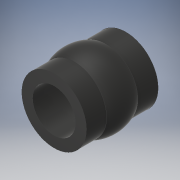
# Autodesk Inventor part: タミヤダンパー部品8.1
Saved by Autodesk Inventor 2020.1 (Build 241239000, 239)
## iProperties
Created: 2018-09-17
Part Number: タミヤダンパー部品8.1
Material: アセタール樹脂、黒
Document SubType Name: Modeling
Designer: 杉本　賢二郎
Density: 1.425 g/cm^3
Appearance: 滑らか - 黒
Author: 杉本　賢二郎
Autodesk Inventor part; units mm, degrees
ref_plane "YZ Plane" through (0, 0, 0) normal (1, 0, 0) x (0, 1, 0)
ref_plane "XZ Plane" through (0, 0, 0) normal (0, 1, 0) x (-1, 0, 0)
ref_plane "XY Plane" through (0, 0, 0) normal (0, 0, 1) x (1, 0, 0)
sketch "スケッチ1" plane through (0, 0, 0) normal (0, 0, 1) x (1, 0, 0)
  line L0 (0, 0) -> (0, 2.5)
  line L1 (0, 0) -> (0, -2.5)
  arc A0 (0, 2.5) -> (0, -2.5) centre (0, 0) ccw
  dimension "d0" = 2.5
  dimension "d1" = 2.5
  dimension "d2" = 2.5
  constraints: 4 end point, 2 point on circle, 1 centre point, 1 point on line, 1 vertical
  measures "d0" distance of L0.start L0.end
  measures "d1" distance of L0.start L1.end
  measures "d2" radius of A0
revolve "回転1" add sketch "スケッチ1" angle 360 about axis through (0, 0, 0) along (0, 1, 0)
sketch "スケッチ2" plane through (0, 0, 0) normal (0, 0, 1) x (1, 0, 0)
  circle A0 centre (0, 0) radius 1.5
  circle A1 centre (0, 0) radius 2.25
  dimension "d4" = 3
  dimension "d5" = 4.5
  constraints: 2 centre point, 2 coincident
  measures "d4" diameter of A0
  measures "d5" diameter of A1
extrude "押し出し1" add sketch "スケッチ2" along normal mid plane 5
sketch "スケッチ3" plane through (0, 0, 0) normal (0, 0, 1) x (1, 0, 0)
  circle A0 centre (0, 0) radius 1.5
  constraints: 1 centre point
extrude "押し出し2" cut sketch "スケッチ3" along normal mid plane 5
